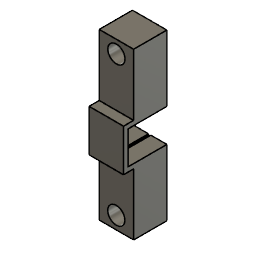
CRAB_Metalens_Holder_FirstVersion (Autodesk Fusion 360 design; units mm, degrees)
part number: 2026-07-09-10-14-52-773
Autodesk Fusion 360 part; units mm, degrees
sketch "Sketch Metalens Holder" plane through (0, 0, 0) normal (1, 0, 0) x (0, 0, -1)
  line L0 (0, 8.15) -> (16.5, 8.15)
  line L1 (16.5, 8.15) -> (16.5, -8.35)
  line L2 (16.5, -8.35) -> (0, -8.35)
  line L3 (0, -8.35) -> (0, 8.15)
  dimension "d3" = 16.5
  dimension "d4" = 16.5
  constraint perpendicular L0 L1
  constraint perpendicular L0 L3
  constraint vertical L3
  constraint horizontal L2
  measures "d3" distance of L0.start L0.end
  measures "d4" distance of L0.end L1.end
extrude "Extrude Metalens Holder" add sketch "Sketch Metalens Holder" along normal blind 6
shell "Shell Metalens Holder" thickness 1.1 removed faces 2 at (6, 2.65, -5.5) at (0, 2.65, -5.5)
sketch "Sketch Screwing Parts" plane through (0, 0, 0) normal (1, 0, 0) x (0, 0, -1)
  line L0 (0, -8.35) -> (16.5, -8.35)
  line L1 (3.5, 8.15) -> (18, 8.15)
  line L2 (18, 8.15) -> (18, 35.85)
  line L3 (18, 35.85) -> (3.5, 35.85)
  line L4 (3.5, 35.85) -> (3.5, 8.15)
  line L5 (3.5, -8.35) -> (18, -8.35)
  line L6 (18, -8.35) -> (18, -36.05)
  line L7 (18, -36.05) -> (3.5, -36.05)
  line L8 (3.5, -36.05) -> (3.5, -8.35)
  line L9 (16.5, -8.35) -> (16.5, 8.15)
  point P0 (0, 8.15)
  dimension "d144" = 3.5
  dimension "d145" = 27.7
  dimension "d148" = 27.7
  dimension "d163" = 1.5
  dimension "d164" = 3.5
  constraint horizontal L1
  constraint vertical L2
  constraint horizontal L3
  constraint vertical L4
  constraint horizontal L5
  constraint vertical L6
  constraint horizontal L7
  constraint vertical L8
  measures "d144" distance of P0 L1.start
  measures "d145" distance of L1.start L3.end
  measures "d148" distance of L5.start L7.end
  measures "d163" distance of L5.end L9
  measures "d164" distance of L0.start L5.start
extrude "Extrude31" add sketch "Sketch Screwing Parts" along normal blind 6
ref_plane "WorkPlane1" through (3, -0.1, -8.25) normal (-1, 0, 0) x (0, 0, 1)
sketch "Sketch Inside Slit" plane through (3, 0, 0) normal (-1, 0, 0) x (0, 0, 1)
  line L0 (-15.4, 7.05) -> (-15.4, -7.25)
  line L1 (-16, 7.65) -> (-0.5, 7.65)
  line L2 (-0.5, 7.65) -> (-0.5, -7.85)
  line L3 (-0.5, -7.85) -> (-16, -7.85)
  line L4 (-16, -7.85) -> (-16, 7.65)
  line L5 (-15.4, 7.05) -> (-1.1, 7.05)
  line L6 (-1.1, 7.05) -> (-1.1, -7.25)
  line L7 (-1.1, -7.25) -> (-15.4, -7.25)
  line L8 (-15.4, -7.25) -> (-15.4, 7.05)
  line L9 (-15.4, 7.05) -> (-16, 7.05)
  line L10 (-1.1, 7.05) -> (-0.5, 7.05)
  line L11 (-1.1, -7.25) -> (-0.5, -7.25)
  line L12 (-15.4, -7.25) -> (-16, -7.25)
  point P0 (-1.1, -7.25)
  point P1 (-1.1, 7.05)
  dimension "d91" = 15.5
  constraint horizontal L1
  constraint vertical L2
  constraint horizontal L3
  constraint vertical L4
  constraint equal L1 L4
  constraint coincident P0 L6.end
  constraint coincident P1 L5.end
  constraint horizontal L5
  constraint vertical L6
  constraint horizontal L7
  constraint vertical L8
  constraint coincident L0.start L5.start
  constraint coincident L4 L9.end
  constraint perpendicular L4 L9
  constraint coincident L2 L10.end
  constraint perpendicular L2 L10
  constraint coincident L2 L11.end
  constraint perpendicular L2 L11
  constraint coincident L0.end L7.end
  constraint coincident L4 L12.end
  constraint perpendicular L4 L12
  measures "d91" distance of L1.start L1.end
extrude "Extrude Inside Slit" cut sketch "Sketch Inside Slit" along normal mid plane 1 contours L2 L6 L10 L11
extrude "Extrude Inside Slit Bis" cut sketch "Sketch Inside Slit" along normal mid plane 1 contours L1 L2 L4 L5 L9 L10
extrude "Extrude Inside Slit BisBis" cut sketch "Sketch Inside Slit" along normal mid plane 1 contours L0 L4 L8 L9 L12
extrude "Extrude Inside Slit BisBisBis" cut sketch "Sketch Inside Slit" along normal mid plane 1
extrude "Extrude" cut 1 faces at (0.8333, 2.2833, -15.4) along direction (0, 0, -1) blind 1.1
extrude "Extrude22" cut 1 faces at (4.3333, 2.2833, -15.4) along direction (0, 0, -1) blind 1.1
extrude "Extrude23" cut 1 faces at (2.8333, -2.4833, -16) along direction (0, 0, -1) blind 0.5
extrude "Extrude24" add 1 faces at (2, -2.85, 0) along direction (0, 0, 1) blind 0.9
extrude "Extrude25" add 2 faces at (2, 8.15, -2.0333) (1.6667, 7.05, -6.2333) along direction (0, 1, 0) blind 0.9
extrude "Extrude26" add 2 faces at (2, -8.35, -2.0333) (4.3333, -7.25, -11.3667) along direction (0, -1, 0) blind 0.9
extrude "Extrude27" add 1 faces at (6, 26.9167, -8.3333) along direction (1, 0, 0) blind 4.5
extrude "Extrude28" add 1 faces at (0, 26.9167, -8.3333) along direction (-1, 0, 0) blind 4.5
extrude "Extrude29" add 1 faces at (-2.1667, 7.6167, -16.5) along direction (0, 0, -1) blind 1.5
extrude "Extrude30" add 1 faces at (-2.1667, -7.8167, -16.5) along direction (0, 0, -1) blind 1.5
sketch "Sketch11" plane through (0, 0, -18) normal (0, 0, -1) x (-1, 0, 0)
  line L0 (4.5, 35.85) -> (-10.5, 35.85)
  line L1 (-10.5, 35.85) -> (-10.5, 7.05)
  line L2 (-10.5, 7.05) -> (-3.5, 7.05)
  line L3 (-3.5, 7.05) -> (-3.5, 7.65)
  line L4 (-3.5, 7.65) -> (-2.5, 7.65)
  line L5 (-2.5, 7.65) -> (-2.5, 7.05)
  line L6 (4.5, 7.05) -> (4.5, 35.85)
  circle A0 centre (-3, 30.3) radius 3.75
  line L7 (-2.5, 7.05) -> (4.5, 7.05)
  dimension "d154" = 7.5
  measures "d154" diameter of A0
extrude "Extrude32" cut sketch "Sketch11" against normal blind 14.5 contours A0
sketch "Sketch12" plane through (0, 0, -18) normal (0, 0, -1) x (-1, 0, 0)
  line L0 (-10.5, -7.25) -> (-10.5, -36.05)
  line L1 (-10.5, -36.05) -> (4.5, -36.05)
  line L2 (4.5, -36.05) -> (4.5, -7.25)
  line L3 (4.5, -7.25) -> (-2.5, -7.25)
  line L4 (-2.5, -7.25) -> (-2.5, -7.85)
  line L5 (-2.5, -7.85) -> (-3.5, -7.85)
  line L6 (-3.5, -7.85) -> (-3.5, -7.25)
  line L7 (-3.5, -7.25) -> (-10.5, -7.25)
  circle A0 centre (-2.9472, -30.4996) radius 3.75
  dimension "d159" = 7.5
  measures "d159" diameter of A0
extrude "Extrude33" cut sketch "Sketch12" against normal blind 14.5 contours A0
